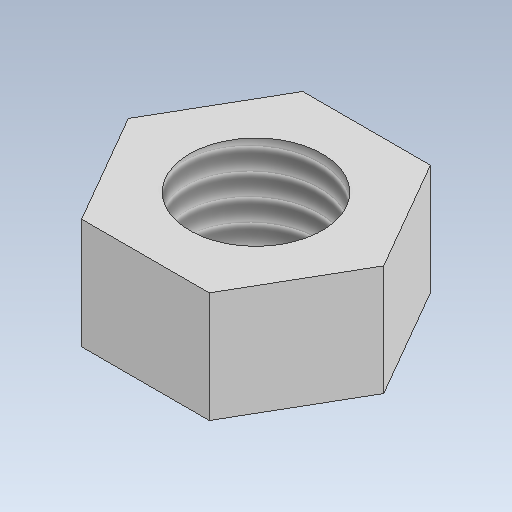
# Autodesk Inventor part: M6_nut_5mm
Saved by Autodesk Inventor 2020.3 (Build 243373000, 373)
## iProperties
Created: 2021-03-23
Part Number: M6_nut_5mm
Material: Ogólny
Document SubType Name: Modeling
Designer: patry
Density: 1 g/cm^3
Appearance: Domyślna
Author: patry
Autodesk Inventor part; units mm, degrees
ref_plane "YZ Plane" through (0, 0, 0) normal (1, 0, 0) x (0, 1, 0)
ref_plane "XZ Plane" through (0, 0, 0) normal (0, 1, 0) x (-1, 0, 0)
ref_plane "XY Plane" through (0, 0, 0) normal (0, 0, 1) x (1, 0, 0)
sketch "Szkic1" plane through (0, 0, 0) normal (0, 1, 0) x (-1, 0, 0)
  line L0 (-2.8868, -5) -> (-5.7735, 0)
  line L1 (-5.7735, 0) -> (-2.8868, 5)
  line L2 (-2.8868, 5) -> (2.8868, 5)
  line L3 (2.8868, 5) -> (5.7735, 0)
  line L4 (5.7735, 0) -> (2.8868, -5)
  line L5 (2.8868, -5) -> (-2.8868, -5)
  circle A0 centre (0, 0) radius 3
  dimension "d0" = 10
  dimension "d1" = 6
  constraints: 12 end point, 2 coincident, 1 centre point, 13 other
  measures "d0" distance between parallel lines of L2 L5
  measures "d1" diameter of A0
extrude "Wyciągnięcie proste1" add sketch "Szkic1" along normal blind 5
thread "Gwint1" size "M6x1" class "6H" standard "ANSI Metric M Profile" length 5
